Autodesk Fusion 360 part; units mm, degrees
(part 2 of 2)
sketch "Skizze13" plane through (0, 0, 25) normal (0, 0, 1) x (-1, 0, 0)
  line L0 (-5.1598, -2.8) -> (-154.8402, -2.8)
  line L1 (-154.8402, -2.8) -> (-157.2, -5.1598)
  line L2 (-157.2, -5.1598) -> (-157.2, -58.8402)
  line L3 (-157.2, -58.8402) -> (-154.8402, -61.2)
  line L4 (-154.8402, -61.2) -> (-5.1598, -61.2)
  line L5 (-5.1598, -61.2) -> (-2.8, -58.8402)
  line L6 (-2.8, -58.8402) -> (-2.8, -5.1598)
  line L7 (-2.8, -5.1598) -> (-5.1598, -2.8)
  line L8 (-6.8, -57.1833) -> (-6.8, -6.8167)
  line L9 (-6.8, -6.8167) -> (-6.8167, -6.8)
  line L10 (-6.8167, -6.8) -> (-153.1833, -6.8)
  line L11 (-153.1833, -6.8) -> (-153.2, -6.8167)
  line L12 (-153.2, -6.8167) -> (-153.2, -57.1833)
  line L13 (-153.2, -57.1833) -> (-153.1833, -57.2)
  line L14 (-153.1833, -57.2) -> (-6.8167, -57.2)
  line L15 (-6.8167, -57.2) -> (-6.8, -57.1833)
  line L16 (-12.9295, -57.2) -> (-153.2, -8.9206)
  line L17 (-147.0705, -6.8) -> (-6.8, -55.0794)
  line L18 (-6.8083, -57.1917) -> (-153.1917, -6.8083) construction
  line L19 (-153.1917, -57.1917) -> (-6.8083, -6.8083) construction
  line L20 (-6.8, -8.9206) -> (-147.0705, -57.2)
  line L21 (-12.9295, -6.8) -> (-153.2, -55.0794)
  dimension "d90" = -4
  dimension "d91" = 4
  dimension "d93" = 2
  dimension "d94" = 4
  dimension "d95" = 2
  constraint coincident L14 L16.start
  constraint coincident L12 L16.end
  constraint coincident L10 L17.start
  constraint coincident L8 L17.end
  constraint parallel L16 L17
  constraint midpoint L15 L18.start
  constraint midpoint L11 L18.end
  constraint midpoint L13 L19.start
  constraint midpoint L9 L19.end
  constraint parallel L16 L18
  constraint coincident L8 L20.start
  constraint coincident L14 L20.end
  constraint parallel L19 L20
  constraint coincident L10 L21.start
  constraint coincident L12 L21.end
  constraint parallel L19 L21
  measures "d91" distance of L16 L17
  measures "d93" distance of L16 L18
  measures "d94" distance of L20 L21
  measures "d95" distance of L19 L20
extrude "Extrusion1'" cut sketch "Skizze13" against normal blind 1 contours L8 L17 L20 | L14 L16 L20 | L10 L17 L21 | L12 L16 L21 bodies 10 in component "Fan Protection"
sketch "Sketch14" plane through (0, 0, 40) normal (0, 0, 1) x (-1, 0, 0)
  line L0 (-156, 0) -> (-160, -4)
  line L1 (-160, -4) -> (-160, -12)
  line L2 (-160, -12) -> (-164, -12)
  line L3 (-164, -12) -> (-168, -16)
  line L4 (-168, -16) -> (-168, -48)
  line L5 (-168, -48) -> (-164, -52)
  line L6 (-164, -52) -> (-160, -52)
  line L7 (-160, -52) -> (-160, -60)
  line L8 (-160, -60) -> (-156, -64)
  line L9 (-156, -64) -> (-4, -64)
  line L10 (-4, -64) -> (0, -60)
  line L11 (0, -60) -> (0, -52)
  line L12 (0, -52) -> (4, -52)
  line L13 (4, -52) -> (8, -48)
  line L14 (8, -48) -> (8, -16)
  line L15 (8, -16) -> (4, -12)
  line L16 (4, -12) -> (0, -12)
  line L17 (0, -12) -> (0, -4)
  line L18 (0, -4) -> (-4, 0)
  line L19 (-4, 0) -> (-156, 0)
  line L20 (-4.7456, -1.8) -> (-1.8, -4.7456)
  line L21 (-1.8, -4.7456) -> (-1.8, -59.2544)
  line L22 (-1.8, -59.2544) -> (-4.7456, -62.2)
  line L23 (-4.7456, -62.2) -> (-155.2544, -62.2)
  line L24 (-155.2544, -62.2) -> (-158.2, -59.2544)
  line L25 (-158.2, -59.2544) -> (-158.2, -4.7456)
  line L26 (-158.2, -4.7456) -> (-155.2544, -1.8)
  line L27 (-155.2544, -1.8) -> (-4.7456, -1.8)
  circle A0 centre (-162.8, -20) radius 2.8
  circle A1 centre (-162.8, -44) radius 2.8
  circle A2 centre (2.8, -44) radius 2.8
  circle A3 centre (2.8, -20) radius 2.8
  circle A4 centre (-67, -57) radius 1.7
  circle A5 centre (-93, -7) radius 1.7
  line L28 (-80, -62.2) -> (-80, -1.8) construction
  circle A6 centre (-80, -59.8) radius 2.4
  circle A7 centre (-80, -59.8) radius 4.2
  line L29 (-75.8, -62.2) -> (-75.8, -59.8)
  line L30 (-84.2, -62.2) -> (-84.2, -59.8)
  arc A8 (-52.9631, -32.9) -> (-42.9, -42.9631) centre (-42, -32) ccw
  line L31 (-72, -62) -> (-12, -62) construction
  line L32 (-12, -62) -> (-12, -2) construction
  line L33 (-12, -2) -> (-72, -2) construction
  line L34 (-72, -2) -> (-72, -62) construction
  line L35 (-72, -62) -> (-12, -2) construction
  line L36 (-12, -62) -> (-72, -2) construction
  line L37 (-80, -32) -> (-1.8, -32) construction
  circle A9 centre (-80, -4.2) radius 4.2
  circle A10 centre (-80, -4.2) radius 2.4
  line L38 (-75.8, -1.8) -> (-75.8, -4.2)
  line L39 (-84.2, -1.8) -> (-84.2, -4.2)
  point P0 (-42, -32)
  dimension "d102" = 4.8
  dimension "d103" = 1.8
  dimension "d104" = 60
  dimension "d105" = 60
  constraint midpoint L23 L28.start
  constraint perpendicular L27 L28
  constraint coincident L28 A6.centre
  constraint tangent L23 A6
  constraint concentric A6 A7
  constraint coincident L23 L29.start
  constraint coincident A7 L29.end
  constraint tangent A7 L29
  constraint coincident L23 L30.start
  constraint coincident A7 L30.end
  constraint tangent A7 L30
  constraint perpendicular L23 L30
  constraint perpendicular L23 L29
  constraint horizontal L31
  constraint perpendicular L31 L32
  constraint parallel L31 L33
  constraint parallel L32 L34
  constraint coincident L35 P0
  constraint coincident L36 P0
  constraint coincident P0 A8.centre
  constraint midpoint L28 L37.start
  constraint midpoint L21 L37.end
  constraint perpendicular L21 L37
  constraint symmetric A6 L37 A10
  constraint symmetric A7 L37 A9
  constraint symmetric L29.start L37 L38.start
  constraint symmetric L29.end L37 L38.end
  constraint symmetric L30.start L37 L39.start
  constraint symmetric L30.end L37 L39.end
  measures "d102" diameter of A6
  measures "d103" distance of A6 A7
  measures "d104" distance of L32.end L33.end
  measures "d105" distance of L31.end L32.end
extrude "Extrude2" add sketch "Sketch14" against normal blind 5 contours L27 A9 | L27 A9 L38 | L27 A9 L39 | L23 A7 L29 | L23 A7 L30 | L23 A7 picked at (-83.5834, -4.4479) picked at (-83.5834, -59.5521) bodies 6 in component "Main Body"
sketch "Sketch15" plane through (0, 0, 35) normal (0, 0, -1) x (1, 0, 0)
  line L0 (84.2, -1.8) -> (80, -1.8)
  circle A0 centre (80, -4.2) radius 2.4
  line L1 (80, -1.8) -> (75.8, -1.8)
  line L2 (75.8, -1.8) -> (75.8, -4.2)
  arc A1 (75.8, -4.2) -> (84.2, -4.2) centre (80, -4.2) ccw
  line L3 (84.2, -4.2) -> (84.2, -1.8)
  circle A2 centre (80, -59.8) radius 2.4
  line L4 (80, -62.2) -> (84.2, -62.2)
  line L5 (84.2, -62.2) -> (84.2, -59.8)
  arc A3 (84.2, -59.8) -> (75.8, -59.8) centre (80, -59.8) ccw
  line L6 (75.8, -59.8) -> (75.8, -62.2)
  line L7 (75.8, -62.2) -> (80, -62.2)
  circle A4 centre (80, -59.8) radius 2.4
extrude "Extrude3" add sketch "Sketch15" along normal blind 1.8 contours A0 | L0 L1 L2 A1 L3 | A2 A4 | L4 L5 A3 L6 L7 bodies 6 in component "Main Body"
chamfer "Chamfer2" distance 6.599 angle 45 2 edges at (80, 62.2, 33.2) (80, 1.8, 33.2) on bodies 6 in component "Main Body"
fillet "Fillet1" radius 4 4 edges at (84.2, 62.2, 33.3005) (75.8, 62.2, 33.3005) (75.8, 1.8, 33.3005) (84.2, 1.8, 33.3005) on bodies 6 in component "Main Body"
sketch "Sketch16" plane through (0, 0, 40) normal (0, 0, 1) x (-1, 0, 0)
  circle A0 centre (-80, -59.8) radius 2.4
  circle A1 centre (-80, -4.2) radius 2.4
  circle A2 centre (-162.8, -20) radius 2.8
  circle A3 centre (-162.8, -44) radius 2.8
  circle A4 centre (2.8, -44) radius 2.8
  circle A5 centre (2.8, -20) radius 2.8
  arc A6 (-75.8807, -58.9805) -> (-84.1193, -58.9805) centre (-80, -59.8) ccw
  arc A7 (-88.0424, -62.2) -> (-84.1193, -58.9805) centre (-88.0424, -58.2) ccw
  line L0 (-88.0424, -62.2) -> (-155.2544, -62.2)
  line L1 (-155.2544, -62.2) -> (-158.2, -59.2544)
  line L2 (-158.2, -59.2544) -> (-158.2, -4.7456)
  line L3 (-158.2, -4.7456) -> (-155.2544, -1.8)
  line L4 (-155.2544, -1.8) -> (-88.0424, -1.8)
  arc A8 (-84.1193, -5.0195) -> (-88.0424, -1.8) centre (-88.0424, -5.8) ccw
  arc A9 (-84.1193, -5.0195) -> (-75.8807, -5.0195) centre (-80, -4.2) ccw
  arc A10 (-71.9576, -1.8) -> (-75.8807, -5.0195) centre (-71.9576, -5.8) ccw
  line L5 (-71.9576, -1.8) -> (-4.7456, -1.8)
  line L6 (-4.7456, -1.8) -> (-1.8, -4.7456)
  line L7 (-1.8, -4.7456) -> (-1.8, -59.2544)
  line L8 (-1.8, -59.2544) -> (-4.7456, -62.2)
  line L9 (-4.7456, -62.2) -> (-71.9576, -62.2)
  arc A11 (-75.8807, -58.9805) -> (-71.9576, -62.2) centre (-71.9576, -58.2) ccw
  line L10 (-4, -64) -> (0, -60)
  line L11 (0, -60) -> (0, -52)
  line L12 (0, -52) -> (4, -52)
  line L13 (4, -52) -> (8, -48)
  line L14 (8, -48) -> (8, -16)
  line L15 (8, -16) -> (4, -12)
  line L16 (4, -12) -> (0, -12)
  line L17 (0, -12) -> (0, -4)
  line L18 (0, -4) -> (-4, 0)
  line L19 (-4, 0) -> (-156, 0)
  line L20 (-156, 0) -> (-160, -4)
  line L21 (-160, -4) -> (-160, -12)
  line L22 (-160, -12) -> (-164, -12)
  line L23 (-164, -12) -> (-168, -16)
  line L24 (-168, -16) -> (-168, -48)
  line L25 (-168, -48) -> (-164, -52)
  line L26 (-164, -52) -> (-160, -52)
  line L27 (-160, -52) -> (-160, -60)
  line L28 (-160, -60) -> (-156, -64)
  line L29 (-156, -64) -> (-4, -64)
  line L30 (-75.8807, 0) -> (-75.8807, -5.0195)
  line L31 (-75.8807, -5.0195) -> (-72.0807, -5.0195)
  line L32 (-72.0807, -5.0195) -> (-72.0807, 0)
  dimension "d113" = 3.8
  constraint vertical L30
  constraint coincident A9.end A10.end
  constraint perpendicular L30 L31
  constraint coincident L19 L32.end
  constraint perpendicular L19 L32
  measures "d113" distance of A9.end L31.end
extrude "Extrude4" cut sketch "Sketch16" against normal blind 4 contours A10 L19 L30 L32 bodies 6 in component "Main Body"
fillet "Fillet2" radius 0.8 4 edges at (75.8807, 2.5098, 36) (72.0807, 0.9009, 36) (75.8807, 2.5098, 40) (72.0807, 0.9009, 40) on bodies 6 in component "Main Body"
sketch "Sketch17" plane through (0, 0, 41.8) normal (0, 0, 1) x (-1, 0, 0)
  circle A0 centre (-143, -57) radius 1.7
  arc A1 (-134.9762, -32.9) -> (-118.9, -48.9762) centre (-118, -32) ccw
  line L0 (-118.9, -48.9762) -> (-118.9, -52.9807)
  arc A2 (-138.9807, -32.9) -> (-118.9, -52.9807) centre (-118, -32) ccw
  line L1 (-138.9807, -32.9) -> (-134.9762, -32.9)
  arc A3 (-118.9, -21.0369) -> (-128.9631, -31.1) centre (-118, -32) ccw
  line L2 (-128.9631, -31.1) -> (-132.973, -31.1)
  arc A4 (-118.9, -17.027) -> (-132.973, -31.1) centre (-118, -32) ccw
  line L3 (-118.9, -17.027) -> (-118.9, -21.0369)
  line L4 (-107.0369, -32.9) -> (-103.027, -32.9)
  arc A5 (-117.1, -46.973) -> (-103.027, -32.9) centre (-118, -32) ccw
  line L5 (-117.1, -46.973) -> (-117.1, -42.9631)
  arc A6 (-117.1, -42.9631) -> (-107.0369, -32.9) centre (-118, -32) ccw
  line L6 (-42.9, -48.9762) -> (-42.9, -52.9807)
  arc A7 (-62.9807, -32.9) -> (-42.9, -52.9807) centre (-42, -32) ccw
  line L7 (-62.9807, -32.9) -> (-58.9762, -32.9)
  arc A8 (-58.9762, -32.9) -> (-42.9, -48.9762) centre (-42, -32) ccw
  line L8 (-42.9, -42.9631) -> (-42.9, -46.973)
  arc A9 (-56.973, -32.9) -> (-42.9, -46.973) centre (-42, -32) ccw
  line L9 (-56.973, -32.9) -> (-52.9631, -32.9)
  arc A10 (-52.9631, -32.9) -> (-42.9, -42.9631) centre (-42, -32) ccw
  line L10 (-41.1, -9.0176) -> (-41.1, -4.0145)
  arc A11 (-14.0145, -31.1) -> (-41.1, -4.0145) centre (-42, -32) ccw
  line L11 (-14.0145, -31.1) -> (-19.0176, -31.1)
  arc A12 (-19.0176, -31.1) -> (-41.1, -9.0176) centre (-42, -32) ccw
  line L12 (-41.1, -15.0238) -> (-41.1, -11.0193)
  arc A13 (-21.0193, -31.1) -> (-41.1, -11.0193) centre (-42, -32) ccw
  line L13 (-21.0193, -31.1) -> (-25.0238, -31.1)
  arc A14 (-25.0238, -31.1) -> (-41.1, -15.0238) centre (-42, -32) ccw
  arc A15 (-41.1, -42.9631) -> (-31.0369, -32.9) centre (-42, -32) ccw
  line L14 (-31.0369, -32.9) -> (-27.027, -32.9)
  arc A16 (-41.1, -46.973) -> (-27.027, -32.9) centre (-42, -32) ccw
  line L15 (-41.1, -46.973) -> (-41.1, -42.9631)
  arc A17 (-41.1, -54.9824) -> (-19.0176, -32.9) centre (-42, -32) ccw
  line L16 (-19.0176, -32.9) -> (-14.0145, -32.9)
  arc A18 (-41.1, -59.9855) -> (-14.0145, -32.9) centre (-42, -32) ccw
  line L17 (-41.1, -59.9855) -> (-41.1, -54.9824)
  arc A19 (-95.0176, -31.1) -> (-117.1, -9.0176) centre (-118, -32) ccw
  line L18 (-117.1, -9.0176) -> (-117.1, -4.0145)
  arc A20 (-90.0145, -31.1) -> (-117.1, -4.0145) centre (-118, -32) ccw
  line L19 (-90.0145, -31.1) -> (-95.0176, -31.1)
  arc A21 (-118.9, -15.0238) -> (-134.9762, -31.1) centre (-118, -32) ccw
  line L20 (-134.9762, -31.1) -> (-138.9807, -31.1)
  arc A22 (-118.9, -11.0193) -> (-138.9807, -31.1) centre (-118, -32) ccw
  line L21 (-118.9, -11.0193) -> (-118.9, -15.0238)
  arc A23 (-128.9631, -32.9) -> (-118.9, -42.9631) centre (-118, -32) ccw
  line L22 (-118.9, -42.9631) -> (-118.9, -46.973)
  arc A24 (-132.973, -32.9) -> (-118.9, -46.973) centre (-118, -32) ccw
  line L23 (-132.973, -32.9) -> (-128.9631, -32.9)
  circle A25 centre (-17, -7) radius 1.7
  circle A26 centre (-93, -7) radius 1.7
  arc A27 (-118.9, -9.0176) -> (-140.9824, -31.1) centre (-118, -32) ccw
  line L24 (-140.9824, -31.1) -> (-145.9855, -31.1)
  arc A28 (-118.9, -4.0145) -> (-145.9855, -31.1) centre (-118, -32) ccw
  line L25 (-118.9, -4.0145) -> (-118.9, -9.0176)
  arc A29 (-107.0369, -31.1) -> (-117.1, -21.0369) centre (-118, -32) ccw
  line L26 (-117.1, -21.0369) -> (-117.1, -17.027)
  arc A30 (-103.027, -31.1) -> (-117.1, -17.027) centre (-118, -32) ccw
  line L27 (-103.027, -31.1) -> (-107.0369, -31.1)
  line L28 (-101.0238, -32.9) -> (-97.0193, -32.9)
  arc A31 (-117.1, -52.9807) -> (-97.0193, -32.9) centre (-118, -32) ccw
  line L29 (-117.1, -52.9807) -> (-117.1, -48.9762)
  arc A32 (-117.1, -48.9762) -> (-101.0238, -32.9) centre (-118, -32) ccw
  line L30 (-42.9, -54.9824) -> (-42.9, -59.9855)
  arc A33 (-69.9855, -32.9) -> (-42.9, -59.9855) centre (-42, -32) ccw
  line L31 (-69.9855, -32.9) -> (-64.9824, -32.9)
  arc A34 (-64.9824, -32.9) -> (-42.9, -54.9824) centre (-42, -32) ccw
  line L32 (-52.9631, -31.1) -> (-56.973, -31.1)
  arc A35 (-42.9, -17.027) -> (-56.973, -31.1) centre (-42, -32) ccw
  line L33 (-42.9, -17.027) -> (-42.9, -21.0369)
  arc A36 (-42.9, -21.0369) -> (-52.9631, -31.1) centre (-42, -32) ccw
  line L34 (-64.9824, -31.1) -> (-69.9855, -31.1)
  arc A37 (-42.9, -4.0145) -> (-69.9855, -31.1) centre (-42, -32) ccw
  line L35 (-42.9, -4.0145) -> (-42.9, -9.0176)
  arc A38 (-42.9, -9.0176) -> (-64.9824, -31.1) centre (-42, -32) ccw
  line L36 (-41.1, -21.0369) -> (-41.1, -17.027)
  arc A39 (-27.027, -31.1) -> (-41.1, -17.027) centre (-42, -32) ccw
  line L37 (-27.027, -31.1) -> (-31.0369, -31.1)
  arc A40 (-31.0369, -31.1) -> (-41.1, -21.0369) centre (-42, -32) ccw
  arc A41 (-41.1, -48.9762) -> (-25.0238, -32.9) centre (-42, -32) ccw
  line L38 (-25.0238, -32.9) -> (-21.0193, -32.9)
  arc A42 (-41.1, -52.9807) -> (-21.0193, -32.9) centre (-42, -32) ccw
  line L39 (-41.1, -52.9807) -> (-41.1, -48.9762)
  line L40 (-95.0176, -32.9) -> (-90.0145, -32.9)
  arc A43 (-117.1, -59.9855) -> (-90.0145, -32.9) centre (-118, -32) ccw
  line L41 (-117.1, -59.9855) -> (-117.1, -54.9824)
  arc A44 (-117.1, -54.9824) -> (-95.0176, -32.9) centre (-118, -32) ccw
  arc A45 (-101.0238, -31.1) -> (-117.1, -15.0238) centre (-118, -32) ccw
  line L42 (-117.1, -15.0238) -> (-117.1, -11.0193)
  arc A46 (-97.0193, -31.1) -> (-117.1, -11.0193) centre (-118, -32) ccw
  line L43 (-97.0193, -31.1) -> (-101.0238, -31.1)
  arc A47 (-140.9824, -32.9) -> (-118.9, -54.9824) centre (-118, -32) ccw
  line L44 (-118.9, -54.9824) -> (-118.9, -59.9855)
  arc A48 (-145.9855, -32.9) -> (-118.9, -59.9855) centre (-118, -32) ccw
  line L45 (-145.9855, -32.9) -> (-140.9824, -32.9)
  circle A49 centre (-67, -57) radius 1.7
  line L46 (-58.9762, -31.1) -> (-62.9807, -31.1)
  arc A50 (-42.9, -11.0193) -> (-62.9807, -31.1) centre (-42, -32) ccw
  line L47 (-42.9, -11.0193) -> (-42.9, -15.0238)
  arc A51 (-42.9, -15.0238) -> (-58.9762, -31.1) centre (-42, -32) ccw
  circle A52 centre (2.8, -20) radius 1.7
  circle A53 centre (2.8, -44) radius 1.7
  circle A54 centre (-162.8, -20) radius 1.7
  circle A55 centre (-162.8, -44) radius 1.7
  line L48 (-156, -64) -> (-4, -64)
  line L49 (-4, -64) -> (0, -60)
  line L50 (0, -60) -> (0, -52)
  line L51 (0, -52) -> (4, -52)
  line L52 (4, -52) -> (8, -48)
  line L53 (8, -48) -> (8, -16)
  line L54 (8, -16) -> (4, -12)
  line L55 (4, -12) -> (0, -12)
  line L56 (0, -12) -> (0, -4)
  line L57 (0, -4) -> (-4, 0)
  line L58 (-4, 0) -> (-156, 0)
  line L59 (-156, 0) -> (-160, -4)
  line L60 (-160, -4) -> (-160, -12)
  line L61 (-160, -12) -> (-164, -12)
  line L62 (-164, -12) -> (-168, -16)
  line L63 (-168, -16) -> (-168, -48)
  line L64 (-168, -48) -> (-164, -52)
  line L65 (-164, -52) -> (-160, -52)
  line L66 (-160, -52) -> (-160, -60)
  line L67 (-160, -60) -> (-156, -64)
  circle A56 centre (-80, -59.8) radius 2.4
  circle A57 centre (-80, -4.2) radius 2.4
  circle A58 centre (-80, -59.8) radius 1.7
  circle A59 centre (-80, -4.2) radius 1.7
  dimension "d118" = 3.4
  constraint concentric A56 A58
  constraint concentric A57 A59
  constraint equal A58 A59
  measures "d118" diameter of A58
extrude "Extrude1" cut sketch "Sketch17" against normal blind 1.8 contours A58 | A59 bodies 8 in component "Back Cover"
chamfer "Chamfer3" distance 0.4 angle 45 2 edges at (82.2376, 60.6679, 40) (82.2376, 5.0679, 40) on bodies 6 in component "Main Body"
component "Main Body" placed x (1, 0, 0) y (0, 1, 0) z (0, 0, 1) at (0, 0, 0)
component "Inside Cover" placed x (1, 0, 0) y (0, 1, 0) z (0, 0, 1) at (0, 0, 0)
component "Back Cover" placed x (1, 0, 0) y (0, 1, 0) z (0, 0, 1) at (0, 0, 0)
component "Fan Protection" placed x (1, 0, 0) y (0, 1, 0) z (0, 0, 1) at (0, 0, 0)
equation "d27 = -1.8 mm - 4 mm"
equation "d42 = -10.60 mm + 1.2 mm"
named bodies: "Main Body", "Inside Cover", "Back Cover"
